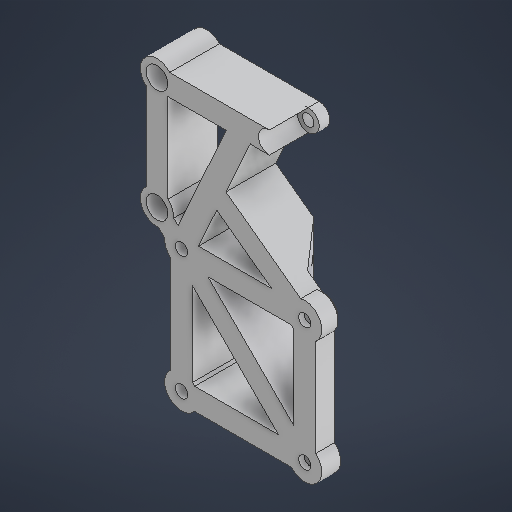
# Autodesk Inventor part: hemera-mount
Saved by Autodesk Inventor 2025 (Build 290162000, 162)
## iProperties
Created: 2024-07-16
Part Number: hemera-mount
Material: Generic
Document SubType Name: Modeling
Designer: Windows 7 was better
Density: 1 g/cm^3
Appearance: Default
Author: Windows 7 was better
Autodesk Inventor part; units mm, degrees
ref_plane "YZ Plane" through (0, 0, 0) normal (1, 0, 0) x (0, 1, 0)
ref_plane "XZ Plane" through (0, 0, 0) normal (0, 1, 0) x (-1, 0, 0)
sketch "Sketch1" plane through (0, 0, 0) normal (0, 0, 1) x (1, 0, 0)
  circle A0 centre (-7, 39.4) radius 1.6 projected
  arc A1 (22.5, 38.8432) -> (22.5, 39.9568) centre (24, 39.4) ccw projected
  circle A2 centre (-7, 8.4) radius 1.6 projected
  circle A3 centre (-0.2171, 1.8572) radius 1.7 projected
  circle A4 centre (-0.2171, -32.1428) radius 1.7 projected
  circle A5 centre (33.7829, -32.1428) radius 1.7 projected
  circle A6 centre (33.7829, 1.8572) radius 1.7 projected
  line L0 (24, 39.4) -> (-7, 39.4) construction
  line L1 (-7, 39.4) -> (-7, 8.4) construction
  line L2 (-7, 8.4) -> (-0.2171, 1.8572) construction
  line L3 (-0.2171, 1.8572) -> (-0.2171, -32.1428) construction
  line L4 (-0.2171, -32.1428) -> (33.7829, -32.1428) construction
  line L5 (33.7829, -32.1428) -> (33.7829, 1.8572) construction
  line L6 (33.7829, 1.8572) -> (-0.2171, 1.8572) construction
  line L7 (16.7829, 39.4) -> (-0.2171, 1.8572) construction
  line L8 (33.7829, 1.8572) -> (8.2829, 20.6286) construction
  line L9 (33.7829, -32.1428) -> (-0.2171, 1.8572) construction
  circle A7 centre (-7, 39.4) radius 4.6
  arc A8 (19.6875, 37.7993) -> (19.6875, 41.0007) centre (24, 39.4) ccw
  arc A9 (19.6875, 41.0007) -> (19.6875, 37.7993) centre (24, 39.4) ccw
  circle A10 centre (-7, 8.4) radius 4.6
  circle A11 centre (-0.2171, 1.8572) radius 4.7
  circle A12 centre (33.7829, 1.8572) radius 4.7
  circle A13 centre (33.7829, -32.1428) radius 4.7
  circle A14 centre (-0.2171, -32.1428) radius 4.7
  line L10 (24, 42.4) -> (-7, 42.4)
  line L11 (-7, 42.4) -> (-7, 36.4)
  line L12 (-7, 36.4) -> (24, 36.4)
  line L13 (24, 36.4) -> (24, 42.4)
  line L14 (24, 42.4) -> (-7, 36.4) construction
  line L15 (-7, 42.4) -> (24, 36.4) construction
  line L16 (-10, 39.4) -> (-10, 8.4)
  line L17 (-10, 8.4) -> (-4, 8.4)
  line L18 (-4, 8.4) -> (-4, 39.4)
  line L19 (-4, 39.4) -> (-10, 39.4)
  line L20 (-10, 39.4) -> (-4, 8.4) construction
  line L21 (-10, 8.4) -> (-4, 39.4) construction
  line L22 (-2.95, 3.0947) -> (14.05, 40.6375)
  line L23 (14.05, 40.6375) -> (19.5158, 38.1625)
  line L24 (19.5158, 38.1625) -> (2.5158, 0.6197)
  line L25 (2.5158, 0.6197) -> (-2.95, 3.0947)
  line L26 (-2.95, 3.0947) -> (19.5158, 38.1625) construction
  line L27 (14.05, 40.6375) -> (2.5158, 0.6197) construction
  line L28 (35.5614, 4.2732) -> (10.0614, 23.0446)
  line L29 (10.0614, 23.0446) -> (6.5044, 18.2126)
  line L30 (6.5044, 18.2126) -> (32.0044, -0.5588)
  line L31 (32.0044, -0.5588) -> (35.5614, 4.2732)
  line L32 (35.5614, 4.2732) -> (6.5044, 18.2126) construction
  line L33 (10.0614, 23.0446) -> (32.0044, -0.5588) construction
  line L34 (-0.2171, 4.8572) -> (33.7829, 4.8572)
  line L35 (33.7829, 4.8572) -> (33.7829, -1.1428)
  line L36 (33.7829, -1.1428) -> (-0.2171, -1.1428)
  line L37 (-0.2171, -1.1428) -> (-0.2171, 4.8572)
  line L38 (-0.2171, 4.8572) -> (33.7829, -1.1428) construction
  line L39 (33.7829, 4.8572) -> (-0.2171, -1.1428) construction
  line L40 (36.7829, 1.8572) -> (36.7829, -32.1428)
  line L41 (36.7829, -32.1428) -> (30.7829, -32.1428)
  line L42 (30.7829, -32.1428) -> (30.7829, 1.8572)
  line L43 (30.7829, 1.8572) -> (36.7829, 1.8572)
  line L44 (36.7829, 1.8572) -> (30.7829, -32.1428) construction
  line L45 (36.7829, -32.1428) -> (30.7829, 1.8572) construction
  line L46 (-0.2171, -35.1428) -> (33.7829, -35.1428)
  line L47 (33.7829, -35.1428) -> (33.7829, -29.1428)
  line L48 (33.7829, -29.1428) -> (-0.2171, -29.1428)
  line L49 (-0.2171, -29.1428) -> (-0.2171, -35.1428)
  line L50 (-0.2171, -35.1428) -> (33.7829, -29.1428) construction
  line L51 (33.7829, -35.1428) -> (-0.2171, -29.1428) construction
  line L52 (-3.2171, -32.1428) -> (-3.2171, 1.8572)
  line L53 (-3.2171, 1.8572) -> (2.7829, 1.8572)
  line L54 (2.7829, 1.8572) -> (2.7829, -32.1428)
  line L55 (2.7829, -32.1428) -> (-3.2171, -32.1428)
  line L56 (-3.2171, -32.1428) -> (2.7829, 1.8572) construction
  line L57 (-3.2171, 1.8572) -> (2.7829, -32.1428) construction
  line L58 (-4.8998, 10.5424) -> (1.8656, 4.0164)
  line L59 (1.8656, 4.0164) -> (-2.2999, -0.302)
  line L60 (-2.2999, -0.302) -> (-9.0653, 6.224)
  line L61 (-9.0653, 6.224) -> (-4.8998, 10.5424)
  line L62 (-4.8998, 10.5424) -> (-2.2999, -0.302) construction
  line L63 (1.8656, 4.0164) -> (-9.0653, 6.224) construction
  line L64 (1.9042, 3.9785) -> (35.9042, -30.0215)
  line L65 (35.9042, -30.0215) -> (31.6616, -34.2641)
  line L66 (31.6616, -34.2641) -> (-2.3384, -0.2641)
  line L67 (-2.3384, -0.2641) -> (1.9042, 3.9785)
  line L68 (1.9042, 3.9785) -> (31.6616, -34.2641) construction
  line L69 (35.9042, -30.0215) -> (-2.3384, -0.2641) construction
  circle A15 centre (24, 39.4) radius 1.6 projected
  point P0 (0, 0)
  point P1 (8.5, 39.4)
  point P2 (-7, 23.9)
  point P3 (21.0329, 11.2429)
  point P4 (16.7829, 1.8572)
  point P5 (33.7829, -15.1428)
  point P6 (16.7829, -32.1428)
  point P7 (-0.2171, -15.1428)
  point P8 (-3.5998, 5.1202)
  point P9 (-10, 11.8871)
  point P10 (-6.573, 3.8199)
  point P11 (-4.9039, 2.2098)
  point P12 (-3.2171, -1.7608)
  point P13 (-3.2171, -28.5248)
  point P14 (3.4009, -35.1428)
  point P15 (30.1649, -35.1428)
  point P16 (36.7829, -28.5248)
  point P17 (36.7829, -1.7608)
  point P18 (32.6477, 6.4181)
  point P19 (12.0179, 21.6043)
  point P20 (18.7177, 36.4)
  point P21 (20.5129, 36.4)
  point P22 (20.5129, 42.4)
  point P23 (-3.5129, 42.4)
  point P24 (-10, 35.9129)
  point P25 (9.4877, 16.0165)
  point P26 (24.6471, 4.8572)
  point P27 (4.4346, 4.8572)
  point P28 (3.4009, -1.1428)
  point P29 (30.1649, -1.1428)
  point P30 (30.7829, -1.7608)
  point P31 (30.7829, -28.5248)
  point P32 (30.1649, -29.1428)
  point P33 (3.4009, -29.1428)
  point P34 (2.7829, -28.5248)
  point P35 (2.7829, -1.7608)
  point P36 (-4, 36.4)
  point P37 (12.1312, 36.4)
  point P38 (-1.1955, 6.9692)
  point P39 (-0.7383, 6.5282)
  point P40 (-1.4576, 6.3906)
  point P41 (-2.4075, 8.1382)
  point P42 (-4, 11.8871)
  point P43 (16.7829, -15.1428)
  point P44 (2.7829, -5.3854)
  point P45 (26.5402, -29.1428)
  point P46 (30.7829, -24.9001)
  point P47 (7.0255, -1.1428)
  dimension "d0" = 3
  dimension "d1" = 3
  dimension "d2" = 3
  dimension "d3" = 3
  dimension "d4" = 3
  dimension "d5" = 3
  dimension "d6" = 3
  dimension "d7" = 6
  dimension "d8" = 6
  dimension "d9" = 6
  dimension "d10" = 6
  dimension "d11" = 6
  dimension "d12" = 6
  dimension "d13" = 6
  dimension "d14" = 6
  dimension "d15" = 6
  dimension "d18" = 6
  constraints: 140 end point, 29 midpoint, 29 parallel, 14 perpendicular, 7 centre point, 4 point on circle, 2 horizontal, 2 point on line, 4 other
  measures "d0" radial gap between concentric circles of A0 A7
  measures "d1" radial gap between concentric circles of A1 A8
  measures "d2" radial gap between concentric circles of A2 A10
  measures "d4" radial gap between concentric circles of A6 A12
  measures "d5" radial gap between concentric circles of A5 A13
  measures "d6" radial gap between concentric circles of A4 A14
  measures "d7" distance of L11.end L10.end
  measures "d8" distance of L17.end L16.end
  measures "d9" distance of L22.end L23.end
  measures "d10" distance of L29.end L28.end
  measures "d11" distance of L34.end L35.end
  measures "d12" distance of L40.end L41.end
  measures "d13" distance of L47.end L46.end
  measures "d14" distance of L52.end L53.end
  measures "d15" distance of L58.end L59.end
  measures "d18" distance of L64.end L65.end
extrude "Extrusion1" add sketch "Sketch1" along normal blind 13.75 contours L19 L18 L12 L11 A0 | A0 L11 L10 A7 L12 L18 L19 | A0 L19 L16 A7 L10 L11 | L11 L12 L18 A7 L16 L19 A0 | L10 A8 A9 L12 L24 L23 L22 A7 | L18 A10 L16 A7 | L10 L13 A1 A15 L12 A8 A9 | A8 L12 L13 A1 L10 | L22 L23 L24 L12 | L12 L24 L28 L29 L30 L34 A11 L58 L22 | L18 L58 L61 A2 L17 L16 A10 | A10 L58 L18 | L16 L17 A2 L61 L60 A10 | L58 A11 L22 | L22 A11 L60 A10 L58 | L58 A10 L60 L61 A2 L17 L18 | L18 L17 A2 L61 L58 | L28 A12 L34 L30 L24 | L24 L30 L29 L28 | L22 L25 A3 L53 L52 L60 A11 | A11 L58 L34 L37 A3 L25 L22 | A11 L34 L58 | L60 L52 A11 | L28 L31 A6 L35 L34 A12 | A12 L40 L43 A6 L31 L28 | L34 L24 A11 | A11 L24 L64 L67 A3 L59 L58 L34 | L58 L59 A3 L37 L34 | L52 L60 L66 A11 | A11 L66 L54 A14 L52 | L52 L53 A3 L67 L60 | L34 L30 A12 L36 L64 A11 L24 | L34 A12 L30 | L34 L35 A6 L43 L42 L30 A12 | A11 L64 L24 | L66 L59 A3 L37 L36 L54 A11 | A11 L54 L66 | L52 L55 A4 L49 L46 A14 | A14 L54 L48 L49 A4 L55 L52 | L67 A3 L59 L60 | L30 L42 L36 A12 | L40 A13 L64 L42 A12 | A12 L42 L36 L35 A6 L43 L40 | L64 A11 L36 L54 L24 | L24 L54 L53 A3 L67 L64 | L54 L36 A11 | A11 L36 L64 L42 A13 L48 L66 L54 | A14 L48 L54 | L46 L49 A4 L55 L54 L48 A14 | A14 L48 L66 A13 L46 | L36 L42 A12 | L42 L43 A6 L31 L30 | L30 L31 A6 L35 L36 L42 | L40 L41 A5 L65 L64 A13 | A13 L46 L47 A5 L41 L40 | L25 L24 L54 L36 L37 A3 | A3 L53 L54 L24 L25 | L64 L36 A11 | L48 A13 L66 | L54 L55 A4 L49 L48 | A13 L66 L65 A5 L47 L46 | L64 A13 L42 | L64 L65 A5 L47 L48 L42 A13 | L48 L42 L41 A5 L65 L66 A13 | A13 L42 L48 | L48 L47 A5 L41 L42
ref_plane "Work Plane1" through (25.5, 25.5, 3.75) normal (-0.7808688, 0, 0.624695) x (0, -1, 0)
sketch "Sketch2" plane through (25.5, 25.5, 3.75) normal (-0.7808688, 0, 0.624695) x (0, -1, 0)
  line L0 (64.6935, -4.8599) -> (10.3184, -4.8599)
  line L1 (10.3184, -4.8599) -> (10.3184, 6.1401)
  line L2 (10.3184, 6.1401) -> (64.6935, 6.1401)
  line L3 (64.6935, 6.1401) -> (64.6935, -4.8599)
  point P0 (25.5, -18.858)
  dimension "d19" = 11
  constraints: 8 end point, 2 parallel, 1 horizontal, 1 perpendicular
  measures "d19" distance of L0.end L1.end
extrude "Extrusion2" cut sketch "Sketch2" against normal blind 22.75
sketch "Sketch3" plane through (0, 0, 0) normal (0, 0, -1) x (-1, 0, 0)
  line L0 (-29.3357, -35.1428) -> (-29.3357, -23.4529) projected
  line L1 (-29.3357, -35.1428) -> (-40.4338, -35.1428)
  line L2 (-40.4338, -35.1428) -> (-40.4338, -38.0174)
  line L3 (-40.4338, -38.0174) -> (-29.3357, -38.0174)
  line L4 (-29.3357, -38.0174) -> (-29.3357, -35.1428)
  line L5 (-40.4338, -35.1428) -> (-29.3357, -35.1428)
  line L6 (-29.3357, -35.1428) -> (-29.3357, 64.8572)
  line L7 (-29.3357, 64.8572) -> (-40.4338, 64.8572)
  line L8 (-40.4338, 64.8572) -> (-40.4338, -35.1428)
  point P0 (0, 0)
  dimension "d40" = 100
  constraints: 16 end point, 4 parallel, 2 horizontal, 2 perpendicular, 1 point on line
  measures "d40" distance of L5.end L6.end
extrude "Extrusion3" cut sketch "Sketch3" against normal up to surface (8.5446 mm away)
chamfer "Chamfer1" distance 0.75 angle 45 1 edges at (37.9773, 3.9779, 8.5446)
sketch "Sketch4" plane through (0, 0, 0) normal (0, 0, -1) x (-1, 0, 0)
  circle A0 centre (-33.7829, -32.1428) radius 1.7 projected
  circle A1 centre (0.2171, -32.1428) radius 1.7 projected
  circle A2 centre (0.2171, 1.8572) radius 1.7 projected
  circle A3 centre (0.2171, -32.1428) radius 3
  circle A4 centre (0.2171, 1.8572) radius 3
  point P0 (0, 0)
  dimension "d27" = 6
  dimension "d28" = 6
  constraints: 2 centre point, 2 coincident
  measures "d27" diameter of A3
  measures "d28" diameter of A4
extrude "Extrusion4" cut sketch "Sketch4" against normal blind 6.75 contours A3 | A4
sketch "Sketch5" plane through (29.3357, -35.1428, 8.5446) normal (0, 0, -1) x (-1, 0, 0)
  circle A0 centre (-4.4472, 3) radius 1.7 projected
  circle A1 centre (-4.4472, 37) radius 1.7 projected
  circle A2 centre (-4.4472, 37) radius 3
  circle A3 centre (-4.4472, 3) radius 3
  point P0 (29.3357, 35.1428)
  dimension "d31" = 6
  dimension "d32" = 6
  constraints: 2 centre point, 2 coincident
  measures "d31" diameter of A2
  measures "d32" diameter of A3
extrude "Extrusion5" cut sketch "Sketch5" against normal blind 3.705
sketch "Sketch6" plane through (0, 0, 13.75) normal (0, 0, 1) x (1, 0, 0)
  circle A0 centre (-7, 8.4) radius 1.6 projected
  circle A1 centre (-7, 39.4) radius 1.6 projected
  circle A2 centre (24, 39.4) radius 1.6 projected
  circle A3 centre (-7, 39.4) radius 3
  circle A4 centre (-7, 8.4) radius 3
  circle A5 centre (24, 39.4) radius 3
  point P0 (0, 0)
  dimension "d35" = 6
  dimension "d36" = 6
  dimension "d37" = 6
  constraints: 3 centre point, 3 coincident
  measures "d35" diameter of A3
  measures "d36" diameter of A4
  measures "d37" diameter of A5
extrude "Extrusion6" cut sketch "Sketch6" against normal blind 10.75 contours A0 | A2 | A3 | A4 | A5
sketch "Sketch7" plane through (0, 0, 13.75) normal (0, 0, 1) x (1, 0, 0)
  circle A0 centre (24, 39.4) radius 1.6 projected
  circle A1 centre (24, 39.4) radius 3
  arc A2 (20.5129, 36.4) -> (20.5129, 42.4) centre (24, 39.4) ccw projected
  circle A3 centre (24, 39.4) radius 4.6
  line L0 (24, 36.4) -> (20.5129, 36.4)
  line L1 (24, 42.4) -> (20.5129, 42.4)
  point P0 (0, 0)
  dimension "d41" = 6
  constraints: 4 end point, 2 centre point, 2 coincident, 2 point on circle, 1 horizontal, 1 tangent
  measures "d41" diameter of A1
extrude "Extrusion7" cut sketch "Sketch7" against normal blind 21.25 contours A1 L1 A2 L0
body "Solid1"
